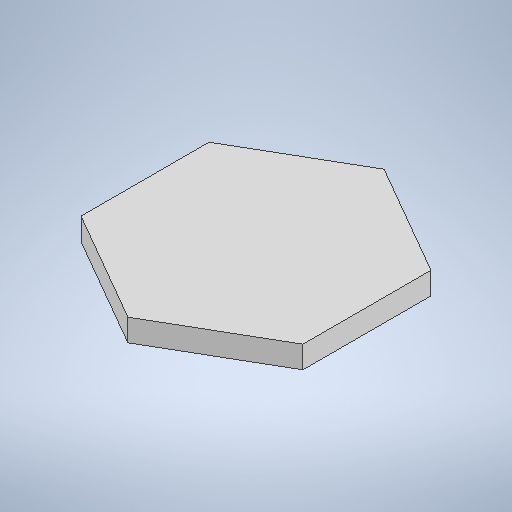
# Autodesk Inventor part: baseBody
Saved by Autodesk Inventor 2025.1 (Build 291241020, 241B)
## iProperties
Created: 2025-03-08
Part Number: baseBody
Material: Generic
Document SubType Name: Modeling
Designer: omiye
Density: 1 g/cm^3
Appearance: Default
Author: omiye
Autodesk Inventor part; units mm, degrees
ref_plane "YZ Plane" through (0, 0, 0) normal (1, 0, 0) x (0, 1, 0)
ref_plane "XZ Plane" through (0, 0, 0) normal (0, 1, 0) x (-1, 0, 0)
ref_plane "XY Plane" through (0, 0, 0) normal (0, 0, 1) x (1, 0, 0)
sketch "Sketch1" plane through (0, 0, 0) normal (0, 1, 0) x (-1, 0, 0)
  line L0 (0, 0) -> (75, 0)
  line L1 (0, 0) -> (75, 0) construction
  line L2 (75, -43.3013) -> (0, -86.6025)
  line L3 (0, -86.6025) -> (-75, -43.3013)
  line L4 (-75, -43.3013) -> (-75, 43.3013)
  line L5 (-75, 43.3013) -> (0, 86.6025)
  line L6 (0, 86.6025) -> (75, 43.3013)
  line L7 (75, 43.3013) -> (75, -43.3013)
  dimension "d0" = 75
  dimension "d1" = 0
  constraints: 16 end point, 2 horizontal, 1 coincident, 1 collinear, 1 midpoint, 13 other
  measures "d0" distance of L0.start L0.end
  measures "d1" distance between parallel lines of L0 L1
extrude "Extrusion1" add sketch "Sketch1" along normal blind 15
body "Solid1"
